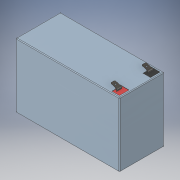
# Autodesk Inventor part: bateria 12mva-7
Saved by Autodesk Inventor 2019.4 (Build 234330000, 330)
## iProperties
Created: 2020-11-16
Part Number: bateria 12mva-7
Material: Plástico PBT
Document SubType Name: Modeling
Designer: Lattes
Density: 1.31 g/cm^3
Appearance: Cinza claro
Author: Lattes
Autodesk Inventor part; units mm, degrees
ref_plane "YZ Plane" through (0, 0, 0) normal (1, 0, 0) x (0, 1, 0)
ref_plane "XZ Plane" through (0, 0, 0) normal (0, 1, 0) x (-1, 0, 0)
ref_plane "XY Plane" through (0, 0, 0) normal (0, 0, 1) x (1, 0, 0)
sketch "Esboço1" plane through (0, 0, 0) normal (0, 1, 0) x (-1, 0, 0)
  line L0 (0, 0) -> (-151, 0)
  line L1 (-151, 0) -> (-151, -65)
  line L2 (-151, -65) -> (0, -65)
  line L3 (0, -65) -> (0, 0)
  dimension "d0" = 151
  dimension "d1" = 65
  constraints: 8 end point, 3 perpendicular, 1 horizontal
  measures "d0" distance of L0.start L0.end
  measures "d1" distance of L0.end L1.end
extrude "Extrusão1" add sketch "Esboço1" along normal blind 94
sketch "Esboço2" plane through (0, 94, 0) normal (0, 1, 0) x (1, 0, 0)
  line L0 (0, 0) -> (151, 0) projected
  line L1 (151, 0) -> (141, 0)
  line L2 (141, 0) -> (141, 6)
  line L3 (141, 6) -> (140.2, 6)
  line L4 (140.2, 6) -> (140.2, 13.8)
  line L5 (140.2, 13.8) -> (141, 13.8)
  line L6 (141, 13.8) -> (141, 6)
  line L7 (151, 0) -> (151, 65) projected
  line L8 (151, 65) -> (141, 65)
  line L9 (151, 65) -> (0, 65) projected
  line L10 (141, 65) -> (141, 59)
  line L11 (141, 59) -> (140.2, 59)
  line L12 (140.2, 59) -> (140.2, 51.2)
  line L13 (140.2, 51.2) -> (141, 51.2)
  line L14 (141, 51.2) -> (141, 59)
  dimension "d4" = 10
  dimension "d5" = 6
  dimension "d6" = 0.8
  dimension "d7" = 7.8
  dimension "d8" = 0.8
  dimension "d9" = 10
  dimension "d10" = 6
  dimension "d11" = 0.8
  dimension "d12" = 7.8
  dimension "d13" = 0.8
  constraints: 24 end point, 6 perpendicular, 4 point on line, 1 collinear
  measures "d4" distance of L0.end L1.end
  measures "d5" distance of L1.end L2.end
  measures "d6" distance of L2.end L3.end
  measures "d7" distance of L3.end L4.end
  measures "d8" distance of L4.end L5.end
  measures "d9" distance of L7.end L8.end
  measures "d10" distance of L8.end L10.end
  measures "d11" distance of L10.end L11.end
  measures "d12" distance of L11.end L12.end
  measures "d13" distance of L12.end L13.end
extrude "Extrusão2" add sketch "Esboço2" along normal blind 3.5
sketch "Esboço3" plane through (140.2, 94, -6) normal (0, 0, 1) x (1, 0, 0)
  line L0 (0, 0) -> (0.8, 0) projected
  line L1 (0.8, 0) -> (-1.2, 0)
  line L2 (-1.2, 4.5) -> (-1.2, 3.5)
  line L3 (0.8, 3.5) -> (0.8, 3.5)
  line L4 (-1.2, 4.5) -> (0.8, 3.5)
  line L5 (0.8, 3.5) -> (0.8, 2.5)
  line L6 (0.8, 2.5) -> (-1.2, 3.5)
  point P0 (-140.2, -94)
  dimension "d16" = 2
  dimension "d17" = 4.5
  dimension "d18" = 1
  dimension "d19" = 1
  constraints: 12 end point, 1 collinear
  measures "d16" distance of L0.end L1.end
  measures "d17" distance of L1.end L2.start
  measures "d18" distance of L2.start L2.end
  measures "d19" distance of L3.end L5.end
sketch "Esboço4" plane through (140.2, 94, -51.2) normal (0, 0, 1) x (1, 0, 0)
  line L0 (0, 0) -> (0.8, 0)
  line L1 (0.8, 0) -> (-1.2, 0)
  line L2 (-1.2, 4.5) -> (-1.2, 3.5)
  line L3 (0.8, 3.5) -> (0.8, 3.5)
  line L4 (-1.2, 4.5) -> (0.8, 3.5)
  line L5 (0.8, 3.5) -> (0.8, 2.5)
  line L6 (0.8, 2.5) -> (-1.2, 3.5)
  point P0 (-140.2, -94)
  point P1 (-140.2, -94)
  dimension "d20" = 2
  dimension "d21" = 4.5
  dimension "d22" = 1
  dimension "d23" = 1
  constraints: 14 end point, 1 collinear
  measures "d20" distance of L0.end L1.end
  measures "d21" distance of L1.end L2.start
  measures "d22" distance of L2.start L2.end
  measures "d23" distance of L3.end L5.end
extrude "Extrusão3" add sketch "Esboço3" against normal blind 7.8
extrude "Extrusão4" add sketch "Esboço4" against normal blind 7.8
sketch "Esboço5" plane through (139, 97.5, -6) normal (-1, 0, 0) x (0, 0, 1)
  line L0 (-3.9, 1) -> (-7.1, 1)
  line L1 (-7.1, 1) -> (-7.1, 0)
  line L2 (-7.1, 0) -> (-0.7, 0)
  line L3 (-0.7, 0) -> (-0.7, 1)
  line L4 (-0.7, 1) -> (-7.1, 1)
  point P0 (6, -97.5)
  point P1 (-7.8, 0)
  point P2 (0, 1)
  point P3 (-7.8, 1)
  dimension "d28" = 3.2
  dimension "d29" = 6.4
  constraints: 10 end point
  measures "d28" distance of L0.start L0.end
  measures "d29" distance of L1.end L2.end
sketch "Esboço6" plane through (141, 97.5, -6) normal (0.4472136, 0.8944272, 0) x (0.8944272, -0.4472136, 0)
  line L0 (-2.2361, 0) -> (-2.2361, 7.8) projected
  line L1 (-2.2361, 0) -> (-2.2361, 7.8)
  line L2 (-2.2361, 3.9) -> (-2.2361, 0.7)
  line L3 (-2.2361, 0.7) -> (-10.2361, 0.7)
  line L4 (-10.2361, 0.7) -> (-10.2361, 7.1)
  line L5 (-10.2361, 7.1) -> (-2.2361, 7.1)
  point P0 (-82.5109, -6)
  dimension "d32" = 3.2
  dimension "d33" = 8
  dimension "d35" = 6.4
  constraints: 10 end point, 2 perpendicular, 2 point on line, 1 collinear, 1 midpoint, 1 vertical
  measures "d32" distance of L2.start L2.end
  measures "d33" distance of L2.end L3.end
  measures "d35" distance of L3.end L4.end
extrude "Extrusão5" add sketch "Esboço6" against normal blind 0.8
sketch "Esboço7" plane through (140.2, 94, -6) normal (0, 0, 1) x (1, 0, 0)
  line L0 (-1.5578, 3.7845) -> (-2.272, 4.1416)
  line L1 (-1.5578, 3.7845) -> (-8.7132, 7.3622) projected
  line L2 (0, 0) -> (0, 2.9) projected
  line L3 (0, 2.9) -> (0, 3.2854)
  line L4 (-2.272, 4.1416) -> (0, 3.0053)
  line L5 (-2.272, 4.1416) -> (0.2683, 4.1416) construction
  line L6 (0, 3.0053) -> (0, 2.9)
  line L7 (-2.272, 4.1416) -> (-2.5664, 3.553)
  line L8 (-2.5664, 3.553) -> (0, 2.2695)
  line L9 (0, 2.2695) -> (0, 3.0053)
  point P0 (-140.2, -94)
  dimension "d38" = 26.57
  constraints: 16 end point, 3 point on line, 2 collinear, 2 perpendicular, 1 equal length, 1 horizontal, 1 vertical
  measures "d38" angle of L4 L5
sketch "Esboço8" plane through (141, 97.5, -51.2) normal (0.4472136, 0.8944272, 0) x (0.8944272, -0.4472136, 0)
  line L0 (-2.2361, 0) -> (-2.2361, 7.8)
  line L1 (-2.2361, 0) -> (-2.2361, 7.8)
  line L2 (-2.2361, 3.9) -> (-2.2361, 0.7)
  line L3 (-2.2361, 0.7) -> (-10.2361, 0.7)
  line L4 (-10.2361, 0.7) -> (-10.2361, 7.1)
  line L5 (-10.2361, 7.1) -> (-2.2361, 7.1)
  point P0 (-82.5109, -51.2)
  point P1 (-82.5109, -6)
  dimension "d39" = 3.2
  dimension "d40" = 8
  dimension "d41" = 6.4
  constraints: 12 end point, 2 perpendicular, 2 point on line, 1 collinear, 1 midpoint, 1 vertical
  measures "d39" distance of L2.start L2.end
  measures "d40" distance of L2.end L3.end
  measures "d41" distance of L3.end L4.end
extrude "Extrusão6" add sketch "Esboço8" against normal blind 0.8
extrude "Extrusão7" cut sketch "Esboço7" against normal blind 100
sketch "Esboço9" plane through (131.8446, 102.0777, -6.7) normal (0, 0, 1) x (0.8944272, -0.4472136, 0)
  line L0 (8, 0) -> (8.4001, -0.8001) projected
  line L1 (8.4001, -0.8001) -> (8, -0.8001)
  line L2 (8, -0.8001) -> (8, 0)
  line L3 (8, 0) -> (8.4001, -0.8001)
  point P0 (-72.2748, -150.2638)
  constraints: 6 end point, 1 collinear, 1 horizontal, 1 perpendicular
sketch "Esboço10" plane through (131.8446, 102.0777, -51.9) normal (0, 0, 1) x (0.8944272, -0.4472136, 0)
  line L0 (8, 0) -> (8.4001, -0.8001)
  line L1 (8.4001, -0.8001) -> (8, -0.8001)
  line L2 (8, -0.8001) -> (8, 0)
  line L3 (8, 0) -> (8.4001, -0.8001)
  point P0 (-72.2748, -150.2638)
  point P1 (-72.2748, -150.2638)
  constraints: 8 end point, 1 collinear, 1 horizontal, 1 perpendicular
extrude "Extrusão8" add sketch "Esboço9" against normal blind 6.4
extrude "Extrusão9" add sketch "Esboço10" against normal blind 6.4
sketch "Esboço11" plane through (141, 97.5, -6) normal (0.4472136, 0.8944272, 0) x (0.8944272, -0.4472136, 0)
  line L0 (-10.2361, 1.7) -> (-9.2361, 0.7)
  line L1 (-10.2361, 1.7) -> (-8.8219, 1.7) construction
  line L2 (-10.2361, 6.1) -> (-9.2361, 7.1)
  line L3 (-10.2361, 6.1) -> (-8.8219, 6.1) construction
  line L4 (-9.2361, 0.7) -> (-10.2361, 0.7)
  line L5 (-10.2361, 0.7) -> (-10.2361, 1.7)
  line L6 (-10.2361, 6.1) -> (-10.2361, 7.1)
  line L7 (-10.2361, 7.1) -> (-9.2361, 7.1)
  line L8 (-7.0361, 4.7) -> (-4.5361, 4.7)
  line L9 (-4.5361, 4.7) -> (-4.5361, 3.1)
  line L10 (-4.5361, 3.1) -> (-7.0361, 3.1)
  line L11 (-7.0361, 3.1) -> (-7.0361, 4.7)
  point P0 (-82.5109, -6)
  dimension "d51" = 4.4
  dimension "d55" = 45
  dimension "d56" = 45
  dimension "d59" = 2.5
  dimension "d60" = 1.6
  dimension "d61" = 2.5
  constraints: 24 end point, 4 perpendicular, 2 equal length, 2 horizontal
  measures "d51" distance of L2.start L0.start
  measures "d55" angle of L0 L1
  measures "d56" angle of L3 L2
  measures "d59" distance of L8.start L8.end
  measures "d60" distance of L8.end L9.end
  measures "d61" distance of L9.end L10.end
sketch "Esboço12" plane through (139, 97.6055, -6.7) normal (0, 0, 1) x (1, 0, 0)
  line L0 (-7.1554, 4.4723) -> (-7.5132, 3.7567) projected
  line L1 (-7.5132, 3.7567) -> (-7.2896, 4.2039)
  line L2 (-7.2896, 4.2039) -> (-6.3952, 3.7567)
  line L3 (-7.2896, 4.2039) -> (-6.8424, 3.9803)
  line L4 (-6.8424, 3.9803) -> (-6.7082, 4.2486)
  line L5 (-7.1554, 4.4723) -> (0, 0.8945) projected
  line L6 (-7.2896, 4.2039) -> (-6.7082, 4.2486)
  point P0 (-139, -97.6055)
  dimension "d52" = 0.5
  dimension "d53" = 1
  dimension "d54" = 0.5
  constraints: 10 end point, 2 perpendicular, 2 point on line, 1 midpoint
  measures "d52" distance of L0.end L1.end
  measures "d53" distance of L1.end L2.end
  measures "d54" distance of L1.end L3.end
sketch "Esboço13" plane through (141, 97.5, -51.2) normal (0.4472136, 0.8944272, 0) x (0.8944272, -0.4472136, 0)
  line L0 (-10.2361, 1.7) -> (-9.2361, 0.7)
  line L1 (-10.2361, 1.7) -> (-8.8219, 1.7) construction
  line L2 (-10.2361, 6.1) -> (-9.2361, 7.1)
  line L3 (-10.2361, 6.1) -> (-8.8219, 6.1) construction
  line L4 (-9.2361, 0.7) -> (-10.2361, 0.7)
  line L5 (-10.2361, 0.7) -> (-10.2361, 1.7)
  line L6 (-10.2361, 6.1) -> (-10.2361, 7.1)
  line L7 (-10.2361, 7.1) -> (-9.2361, 7.1)
  line L8 (-7.0361, 4.7) -> (-4.5361, 4.7)
  line L9 (-4.5361, 4.7) -> (-4.5361, 3.1)
  line L10 (-4.5361, 3.1) -> (-7.0361, 3.1)
  line L11 (-7.0361, 3.1) -> (-7.0361, 4.7)
  point P0 (-82.5109, -51.2)
  point P1 (-82.5109, -6)
  dimension "d62" = 4.4
  dimension "d63" = 45
  dimension "d64" = 45
  dimension "d65" = 2.5
  dimension "d66" = 1.6
  dimension "d67" = 2.5
  constraints: 24 end point, 4 perpendicular, 2 equal length, 2 horizontal
  measures "d62" distance of L2.start L0.start
  measures "d63" angle of L0 L1
  measures "d64" angle of L3 L2
  measures "d65" distance of L8.start L8.end
  measures "d66" distance of L8.end L9.end
  measures "d67" distance of L9.end L10.end
extrude "Extrusão10" cut sketch "Esboço11" against normal blind 0.8
extrude "Extrusão11" cut sketch "Esboço13" against normal blind 0.8
sketch "Esboço14" plane through (139, 97.6055, -6.7) normal (0, 0, 1) x (1, 0, 0)
  line L0 (-7.2225, 4.3381) -> (-6.261, 4.025)
  line L1 (-7.5132, 3.7567) -> (-6.6188, 3.3095) projected
  line L2 (-7.4461, 3.8909) -> (-6.6188, 3.3095)
  line L3 (-7.2225, 4.3381) -> (-7.1554, 4.4723)
  line L4 (-6.261, 4.025) -> (-7.1554, 4.4723)
  line L5 (-7.4461, 3.8909) -> (-7.5132, 3.7567)
  line L6 (-7.5132, 3.7567) -> (-6.6188, 3.3095)
  point P0 (-139, -97.6055)
  dimension "d73" = 0.5
  constraints: 12 end point, 1 collinear, 1 perpendicular
  measures "d73" distance of L0.start L2.start
extrude "Extrusão12" cut sketch "Esboço14" against normal blind 100
fillet "Arredondamento1" radius 2 4 edges at (141, 97.5, -55.1) (141, 97.5, -9.9) (140.2, 97.0053, -9.9) (140.2, 97.0053, -55.1)
fillet "Arredondamento2" radius 1 12 edges at (75.5, 94, 0) (0, 94, -32.5) (75.5, 94, -65) (151, 47, 0) (151, 94, -32.5) (151, 47, -65) (151, 0, -32.5) (75.5, 0, 0) (0, 47, 0) (0, 47, -65) (75.5, 0, -65) (0, 0, -32.5)
sketch "Esboço15" plane through (0, 94, 0) normal (0, 1, 0) x (1, 0, 0)
  line L0 (140.2, 13.8) -> (141, 13.8) projected
  line L1 (141, 13.8) -> (131, 13.8)
  point P0 (0, 0)
  dimension "d78" = 10
  constraints: 2 end point, 1 horizontal
  measures "d78" distance of L0.end L1.end
sketch "Esboço16" plane through (1, 1, 0) normal (0, 0, 1) x (1, 0, 0)
  line L0 (140, 93) -> (140, 95.2639) projected
  line L1 (140, 93) -> (130, 93)
  line L2 (149, 93) -> (0, 93) projected
  line L3 (130, 93) -> (130, 99)
  point P0 (-1, -1)
  dimension "d79" = 10
  dimension "d80" = 6
  constraints: 4 end point, 1 point on line, 1 vertical
  measures "d79" distance of L0.start L1.end
  measures "d80" distance of L1.end L3.end
sketch "Esboço17" plane through (1, 1, 0) normal (0, 0, 1) x (1, 0, 0)
  line L0 (140, 93) -> (140, 95.2639) projected
  line L1 (140, 93) -> (140, 95.2639)
  line L2 (140, 93) -> (130, 93)
  line L3 (149, 93) -> (0, 93) projected
  line L4 (130, 93) -> (130, 99)
  line L5 (130, 99) -> (140, 99)
  line L6 (130, 99) -> (130.5, 99)
  line L7 (140, 93) -> (140, 96.5)
  line L8 (140, 96.5) -> (130, 99)
  line L9 (135, 97.75) -> (134.8059, 96.9739)
  line L10 (135, 97.75) -> (135.8, 97.75) construction
  line L11 (134.8059, 96.9739) -> (130, 98.1757)
  line L12 (130, 98.1757) -> (130.194, 98.9515)
  line L13 (134.8059, 96.9739) -> (140.7545, 95.4864)
  arc A0 (139.2, 94.7694) -> (138.0946, 96.5582) centre (137.2, 94.7694) ccw projected
  line L14 (139.2, 94.7694) -> (139.2, 95.8751)
  line L15 (140, 95.675) -> (137.0896, 96.4028)
  line L16 (139.2, 95.8751) -> (137.0896, 96.4028)
  line L17 (137.0896, 96.4028) -> (137.2837, 97.1791)
  line L18 (139.2, 95.8751) -> (139.2, 93)
  point P0 (-1, -1)
  dimension "d81" = 10
  dimension "d82" = 6
  dimension "d83" = 0.5
  dimension "d84" = 3.5
  dimension "d85" = 0.8
  dimension "d86" = 104.04
  dimension "d87" = 3
  constraints: 34 end point, 10 point on line, 5 perpendicular, 3 vertical, 1 collinear, 1 equal length, 1 horizontal, 1 midpoint, 1 tangent
  measures "d81" distance of L0.start L2.end
  measures "d82" distance of L2.end L4.end
  measures "d83" distance of L4.end L6.end
  measures "d84" distance of L0.start L7.end
  measures "d85" distance of L9.start L9.end
  measures "d86" angle of L9 L10
  measures "d87" distance of L15.start L15.end
sketch "Esboço18" plane through (140.2, 94, -6) normal (0, 0, 1) x (1, 0, 0)
  line L0 (0.8, 0) -> (0.8, 2.2639) projected
  line L1 (0.8, 2.2639) -> (0.8, 0)
  line L2 (0.8, 0) -> (0.8, 3)
  line L3 (-4.4299, 3.7337) -> (-9.2, 5.1648)
  line L4 (-9.2, 5.1648) -> (0, 2.4048)
  line L5 (0, 2.4048) -> (0, 0)
  line L6 (-9.2, 5.1648) -> (-8.9701, 5.931)
  line L7 (-8.9701, 5.931) -> (0.8, 3)
  line L8 (0, 0) -> (0.8, 0)
  line L9 (9.8, 0) -> (-139.2, 0) projected
  line L10 (0.8, 3) -> (0.8, 0)
  point P0 (-140.2, -94)
  point P1 (-1, -1)
  point P2 (-1, -1)
  constraints: 18 end point, 2 collinear, 1 perpendicular, 1 point on line, 1 vertical
sketch "Esboço19" plane through (140.2, 94, -51.2) normal (0, 0, 1) x (1, 0, 0)
  line L0 (0.8, 0) -> (0.8, 2.2639)
  line L1 (0.8, 2.2639) -> (0.8, 0)
  line L2 (0.8, 0) -> (0.8, 3)
  line L3 (-4.4299, 3.7337) -> (-9.2, 5.1648)
  line L4 (-9.2, 5.1648) -> (0, 2.4048)
  line L5 (0, 2.4048) -> (0, 0)
  line L6 (-9.2, 5.1648) -> (-8.9701, 5.931)
  line L7 (-8.9701, 5.931) -> (0.8, 3)
  line L8 (0, 0) -> (0.8, 0)
  line L9 (9.8, 0) -> (-139.2, 0)
  line L10 (0.8, 3) -> (0.8, 0)
  point P0 (-140.2, -94)
  point P1 (-140.2, -94)
  point P2 (-1, -1)
  point P3 (-1, -1)
  constraints: 22 end point, 2 collinear, 1 perpendicular, 1 point on line, 1 vertical
sketch "Esboço20" plane through (140.2, 94, -6) normal (0, 0, 1) x (1, 0, 0)
  line L0 (0, 0) -> (0.8, 0)
  line L1 (9.8, 0) -> (-139.2, 0)
  line L2 (0, 1.7694) -> (-0.1156, 1.7694)
  line L3 (-0.1156, 2.4395) -> (0, 2.4048)
  line L4 (0, 1.7694) -> (0, 2.4048)
  line L5 (0.6399, 3.048) -> (0.6399, 8.7238)
  line L6 (0.6399, 8.7238) -> (-8.9701, 8.7238)
  line L7 (-8.9701, 8.7238) -> (-8.9701, 5.931)
  line L8 (0.6399, 3.048) -> (-8.9701, 5.931)
  line L9 (-0.1156, 2.4395) -> (-0.1156, 1.7694)
  point P0 (-140.2, -94)
  point P1 (-140.2, -94)
  point P2 (-1, -1)
  point P3 (-1, -1)
  constraints: 20 end point, 2 perpendicular, 2 vertical, 1 collinear
extrude "Extrusão13" add sketch "Esboço18" against normal blind 7.8
extrude "Extrusão14" add sketch "Esboço19" against normal blind 7.8
extrude "Extrusão15" cut sketch "Esboço20" against normal blind 100
sketch "Esboço21" plane through (140.2, 94, -6) normal (0, 0, 1) x (1, 0, 0)
  line L0 (-9.2, 5.1648) -> (-8.9701, 5.931) projected
  line L1 (-9.2, 5.1648) -> (-8.9701, 5.931)
  line L2 (-9.0851, 5.5479) -> (-9.0132, 5.7874)
  line L3 (-9.0132, 5.7874) -> (-9.1569, 5.3084)
  line L4 (-9.1569, 5.3084) -> (-8.9551, 5.3084) construction
  line L5 (-8.9701, 5.931) -> (-8.8408, 5.8922)
  line L6 (-8.9701, 5.931) -> (0.8, 3) projected
  line L7 (-8.9701, 5.931) -> (-8.4912, 5.7874)
  line L8 (-9.0132, 5.7874) -> (-8.4912, 5.7874)
  line L9 (-9.2, 5.1648) -> (0, 2.4048) projected
  line L10 (-9.2, 5.1648) -> (-8.7211, 5.0211)
  line L11 (-8.7211, 5.0211) -> (-9.1569, 5.3084)
  point P0 (-140.2, -94)
  dimension "d114" = 0.8
  dimension "d115" = 0.25
  dimension "d116" = 0.5
  dimension "d120" = 0.135
  dimension "d121" = 0.5
  dimension "d122" = 0.5
  constraints: 18 end point, 5 point on line, 1 collinear, 1 horizontal, 1 midpoint
  measures "d114" distance of L0.start L0.end
  measures "d115" distance of L2.start L2.end
  measures "d116" distance of L2.end L3.end
  measures "d120" distance of L0.end L5.end
  measures "d121" distance of L0.end L7.end
  measures "d122" distance of L0.start L10.end
extrude "Extrusão16" cut sketch "Esboço21" against normal blind 100
fillet "Arredondamento3" radius 2 2 edges at (141, 97, -55.1) (141, 97, -9.9)
fillet "Arredondamento4" radius 1 2 edges at (140.2, 96.4048, -55.1) (140.2, 96.4048, -9.9)
sketch "Esboço22" plane through (131.7088, 99.7874, -6) normal (0.2873479, 0.9578263, 0) x (0.9578263, -0.2873479, 0)
  line L0 (-0.5, 0) -> (7.5, 0)
  line L1 (-0.5, 0) -> (-0.5, 0.7)
  line L2 (-0.5, 0.7) -> (7.5, 0.7)
  line L3 (-0.5, 7.8) -> (-0.5, 7.1)
  line L4 (-0.5, 7.1) -> (7.5, 7.1)
  line L5 (7.5, 7.8) -> (-0.5, 7.8)
  line L6 (7.5, 0.7) -> (7.5, 0)
  line L7 (7.5, 7.1) -> (7.5, 7.8)
  point P0 (-97.4805, -6)
  dimension "d127" = 8
  dimension "d128" = 0.7
  dimension "d129" = 0.7
  constraints: 16 end point, 1 collinear, 1 horizontal, 1 vertical
  measures "d127" distance of L0.start L0.end
  measures "d128" distance of L0.start L1.end
  measures "d129" distance of L3.start L3.end
extrude "Extrusão17" cut sketch "Esboço22" against normal blind 0.8
sketch "Esboço23" plane through (131.7088, 99.7874, -51.2) normal (0.2873479, 0.9578263, 0) x (0.9578263, -0.2873479, 0)
  line L0 (-0.5, 0) -> (7.5, 0)
  line L1 (-0.5, 0) -> (-0.5, 0.7)
  line L2 (-0.5, 0.7) -> (7.5, 0.7)
  line L3 (-0.5, 7.8) -> (-0.5, 7.1)
  line L4 (-0.5, 7.1) -> (7.5, 7.1)
  line L5 (7.5, 7.8) -> (-0.5, 7.8)
  line L6 (7.5, 0.7) -> (7.5, 0)
  line L7 (7.5, 7.1) -> (7.5, 7.8)
  point P0 (-97.4805, -51.2)
  point P1 (-97.4805, -6)
  dimension "d132" = 8
  dimension "d133" = 0.7
  dimension "d134" = 0.7
  constraints: 16 end point, 1 collinear, 1 horizontal, 1 vertical
  measures "d132" distance of L0.start L0.end
  measures "d133" distance of L0.start L1.end
  measures "d134" distance of L3.start L3.end
extrude "Extrusão18" cut sketch "Esboço23" against normal blind 0.8
sketch "Esboço24" plane through (139.5747, 97.4276, -6) normal (0.2873479, 0.9578263, 0) x (0.9578263, -0.2873479, 0)
  line L0 (-7.7122, 7.1) -> (-8.7122, 6.1)
  line L1 (-8.7122, 1.7) -> (-7.7122, 0.7)
  line L2 (-5.5122, 4.7) -> (-3.0122, 4.7)
  line L3 (-3.0122, 4.7) -> (-3.0122, 3.1)
  line L4 (-3.0122, 3.1) -> (-5.5122, 3.1)
  line L5 (-5.5122, 3.1) -> (-5.5122, 4.7)
  line L6 (-7.7122, 0.7) -> (-8.7122, 0.7)
  line L7 (-8.7122, 1.7) -> (-8.7122, 0.7)
  line L8 (-8.7122, 6.1) -> (-8.7122, 7.1)
  line L9 (-8.7122, 7.1) -> (-7.7122, 7.1)
  point P0 (-105.6927, -6)
  dimension "d146" = 1.6
  constraints: 20 end point, 3 perpendicular, 1 point on line
  measures "d146" distance of L2.end L3.end
sketch "Esboço25" plane through (139.5747, 97.4276, -51.2) normal (0.2873479, 0.9578263, 0) x (0.9578263, -0.2873479, 0)
  line L0 (-7.7122, 7.1) -> (-8.7122, 6.1)
  line L1 (-8.7122, 1.7) -> (-7.7122, 0.7)
  line L2 (-5.5122, 4.7) -> (-3.0122, 4.7)
  line L3 (-3.0122, 4.7) -> (-3.0122, 3.1)
  line L4 (-3.0122, 3.1) -> (-5.5122, 3.1)
  line L5 (-5.5122, 3.1) -> (-5.5122, 4.7)
  line L6 (-7.7122, 0.7) -> (-8.7122, 0.7)
  line L7 (-8.7122, 1.7) -> (-8.7122, 0.7)
  line L8 (-8.7122, 6.1) -> (-8.7122, 7.1)
  line L9 (-8.7122, 7.1) -> (-7.7122, 7.1)
  point P0 (-105.6927, -51.2)
  point P1 (-105.6927, -6)
  dimension "d147" = 1.6
  constraints: 20 end point, 3 perpendicular, 1 point on line
  measures "d147" distance of L2.end L3.end
extrude "Extrusão19" cut sketch "Esboço24" against normal blind 0.8
extrude "Extrusão20" cut sketch "Esboço25" against normal blind 0.8
fillet "Arredondamento9" radius 0.2 8 edges at (131.1868, 99.7874, -55.1) (131.7088, 99.7874, -55.1) (131.0431, 99.3084, -55.1) (131.7088, 99.7874, -9.9) (131.1868, 99.7874, -9.9) (131.0431, 99.3084, -9.9) (131.4789, 99.0211, -9.9) (131.4789, 99.0211, -55.1)
fillet "Arredondamento10" radius 0.2 36 edges at (131.4798, 99.023, -57.8003) (131.7324, 98.945, -58.0647) (131.0894, 99.3253, -57.3395) (131.1149, 99.5479, -57.3) (131.2162, 99.7478, -57.3395) (131.5075, 99.7874, -57.6072) (131.7085, 99.7852, -57.8003) (131.9623, 99.7113, -58.0647) (131.3109, 99.1319, -57.6072) (131.4798, 99.023, -12.6003) (131.7324, 98.945, -12.8647) (131.0894, 99.3253, -12.1395) (131.1149, 99.5479, -12.1) (131.2162, 99.7478, -12.1395) (131.5075, 99.7874, -12.4072) (131.7085, 99.7852, -12.6003) (131.9623, 99.7113, -12.8647) (131.3109, 99.1319, -12.4072) (131.3109, 99.1319, -52.5928) (131.0894, 99.3253, -52.8605) (131.1149, 99.5479, -52.9) (131.2162, 99.7478, -52.8605) (131.5075, 99.7874, -52.5928) (131.7085, 99.7852, -52.3997) (131.9623, 99.7113, -52.1353) (131.7324, 98.945, -52.1353) (131.4798, 99.023, -52.3997) (131.0894, 99.3253, -7.6605) (131.1149, 99.5479, -7.7) (131.2162, 99.7478, -7.6605) (131.5075, 99.7874, -7.3928) (131.7085, 99.7852, -7.1997) (131.9623, 99.7113, -6.9353) (131.4798, 99.023, -7.1997) (131.7324, 98.945, -6.9353) (131.3109, 99.1319, -7.3928)
fillet "Arredondamento11" radius 0.2 32 edges at (132.2502, 99.5638, -51.9) (132.0728, 99.2606, -51.9) (132.054, 98.9097, -51.9) (135.4457, 97.8311, -51.9) (135.6756, 98.5973, -51.9) (132.2502, 99.5638, -6.7) (132.0728, 99.2606, -6.7) (132.054, 98.9097, -6.7) (135.4457, 97.8311, -6.7) (135.6756, 98.5973, -6.7) (138.7775, 97.2491, -6.7) (138.8925, 97.6323, -6.35) (138.6626, 96.866, -6.35) (138.7775, 97.2491, -51.9) (138.8925, 97.6323, -51.55) (138.6626, 96.866, -51.55) (132.2502, 99.5638, -13.1) (132.0728, 99.2606, -13.1) (132.054, 98.9097, -13.1) (135.4457, 97.8311, -13.1) (135.6756, 98.5973, -13.1) (138.7775, 97.2491, -13.1) (138.8925, 97.6323, -13.45) (138.6626, 96.866, -13.45) (132.2502, 99.5638, -58.3) (132.0728, 99.2606, -58.3) (132.054, 98.9097, -58.3) (135.4457, 97.8311, -58.3) (135.6756, 98.5973, -58.3) (138.7775, 97.2491, -58.3) (138.6626, 96.866, -58.65) (138.8925, 97.6323, -58.65)
fillet "Arredondamento12" radius 0.2 36 edges at (139.3294, 97.5012, -59) (138.9318, 97.5593, -59) (138.7775, 97.2491, -59) (138.7356, 96.9053, -59) (139.1708, 96.7135, -59) (140.0023, 96.2577, -59) (140.2, 94.8304, -59) (141, 94.756, -59) (140.6046, 96.7058, -59) (139.3294, 97.5012, -13.8) (138.9318, 97.5593, -13.8) (138.7775, 97.2491, -13.8) (138.7356, 96.9053, -13.8) (139.1708, 96.7135, -13.8) (140.0023, 96.2577, -13.8) (140.2, 94.8304, -13.8) (141, 94.756, -13.8) (140.6046, 96.7058, -13.8) (141, 94.756, -51.2) (139.3294, 97.5012, -51.2) (138.9318, 97.5593, -51.2) (138.7775, 97.2491, -51.2) (138.7356, 96.9053, -51.2) (139.1708, 96.7135, -51.2) (140.0023, 96.2577, -51.2) (140.2, 94.8304, -51.2) (140.6046, 96.7058, -51.2) (140.6046, 96.7058, -6) (139.3294, 97.5012, -6) (138.9318, 97.5593, -6) (138.7775, 97.2491, -6) (138.7356, 96.9053, -6) (139.1708, 96.7135, -6) (140.0023, 96.2577, -6) (140.2, 94.8304, -6) (141, 94.756, -6)
sketch "Esboço26" plane through (0, 94, 0) normal (0, 1, 0) x (1, 0, 0)
  line L0 (150, 1) -> (1, 1) projected
  line L1 (141, 13.6) -> (141, 6.2) projected
  line L2 (141, 9.9) -> (137, 9.9)
  line L3 (137, 9.9) -> (137, 16.9)
  line L4 (137, 16.9) -> (148, 16.9)
  line L5 (148, 16.9) -> (148, 2.9)
  line L6 (137, 16.9) -> (137, 2.9)
  line L7 (137, 2.9) -> (148, 2.9)
  line L8 (150, 64) -> (151, 64) projected
  line L9 (150, 64) -> (148, 64)
  line L10 (1, 64) -> (150, 64) projected
  line L11 (148, 64) -> (148, 62.1)
  line L12 (148, 62.1) -> (137, 62.1)
  line L13 (137, 62.1) -> (137, 48.1)
  line L14 (137, 48.1) -> (148, 48.1)
  line L15 (148, 48.1) -> (148, 62.1)
  point P0 (0, 0)
  dimension "d165" = 4
  dimension "d166" = 7
  dimension "d167" = 11
  dimension "d168" = 14
  dimension "d170" = 2
  dimension "d171" = 1.9
  dimension "d172" = 11
  dimension "d173" = 14
  dimension "d174" = 11
  constraints: 24 end point, 4 perpendicular, 3 horizontal, 1 midpoint, 1 point on line
  measures "d165" distance of L2.start L2.end
  measures "d166" distance of L2.end L3.end
  measures "d167" distance of L3.end L4.end
  measures "d168" distance of L4.end L5.end
  measures "d170" distance of L8.start L9.end
  measures "d171" distance of L9.end L11.end
  measures "d172" distance of L11.end L12.end
  measures "d173" distance of L12.end L13.end
  measures "d174" distance of L13.end L14.end
extrude "Extrusão21" cut sketch "Esboço26" against normal blind 0.2
fillet "Arredondamento13" radius 0.2 8 edges at (142.5, 93.8, -16.9) (137, 93.8, -9.9) (142.5, 93.8, -62.1) (137, 93.8, -55.1) (142.5, 93.8, -2.9) (148, 93.8, -9.9) (148, 93.8, -55.1) (142.5, 93.8, -48.1)
